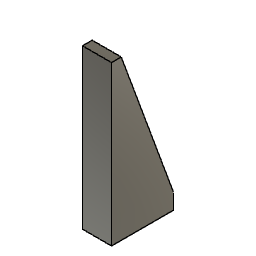
Front Panel Holders v2 (Autodesk Fusion 360 design; units mm, degrees)
Autodesk Fusion 360 part; units mm, degrees
sketch "Sketch1" plane through (0, 0, 0) normal (0, 1, 0) x (1, 0, 0)
  line L0 (0, 0) -> (15, 0)
  line L1 (15, 0) -> (15, -80)
  line L2 (15, -80) -> (0, -80)
  line L3 (0, -80) -> (0, 0)
  dimension "d4" = 15
  dimension "d5" = 80
  constraint horizontal L0
  constraint vertical L1
  constraint horizontal L2
  constraint vertical L3
  constraint coincident L0.start L3.end
  measures "d4" distance of L0.start L0.end
  measures "d5" distance of L0.start L2.end
extrude "Extrude1" add sketch "Sketch1" along normal blind 5
sketch "Sketch3" plane through (0, 5, 0) normal (0, 1, 0) x (-1, 0, 0)
  line L0 (0, 80) -> (-15, 80)
  line L1 (-15, 80) -> (-15, 0)
  line L2 (-15, 0) -> (0, 0)
  line L3 (0, 0) -> (0, 80)
  line L4 (-15, 0) -> (-10, 0)
  line L5 (-10, 0) -> (-10, 8)
  line L6 (-10, 8) -> (-15, 8)
  line L7 (-15, 8) -> (-15, 0)
  dimension "d10" = 5
  dimension "d11" = 8
  constraint horizontal L4
  constraint vertical L5
  constraint horizontal L6
  constraint vertical L7
  constraint coincident L1.end L2.start
  measures "d10" distance of L1.end L4.end
  measures "d11" distance of L1.end L6.end
extrude "Extrude2" add sketch "Sketch3" along normal blind 35 contours L1 L2 L4 L5 L6 L7
sketch "Sketch4" plane through (15, 0, 0) normal (1, 0, 0) x (0, 1, 0)
  line L0 (0, 80) -> (0, 0)
  line L1 (0, 0) -> (40, 0)
  line L2 (40, 0) -> (40, 8)
  line L3 (40, 8) -> (5, 8)
  line L4 (5, 8) -> (5, 80)
  line L5 (5, 80) -> (0, 80)
  line L6 (5, 80) -> (40, 8)
  line L7 (40, 8) -> (5, 8)
  line L8 (5, 8) -> (5, 80)
  constraint coincident L4.end L5.start
  constraint coincident L2.end L3.start
  constraint coincident L3.end L4.start
extrude "Extrude4" add 1 faces at (10, 1.6667, 80) along direction (0, 0, 1) blind 2
extrude "Extrude6" cut 1 faces at (13.3333, 40, 5.3333) along direction (0, -1, 0) blind 8
sketch "Sketch6" plane through (15, 0, 0) normal (1, 0, 0) x (0, 1, 0)
  line L0 (32, 0) -> (32, 8)
  line L1 (32, 8) -> (5, 8)
  line L2 (5, 8) -> (5, 82)
  line L3 (5, 82) -> (0, 82)
  line L4 (0, 82) -> (0, 0)
  line L5 (0, 0) -> (32, 0)
  line L6 (5, 82) -> (5, 8)
  line L7 (5, 8) -> (32, 8)
  line L8 (32, 8) -> (5, 82)
  constraint coincident L2.end L3.start
  constraint coincident L1.end L2.start
  constraint coincident L0.end L1.start
extrude "Extrude7" add sketch "Sketch6" against normal blind 5 contours L1 L2 L6 L7 L8
sketch "Sketch7" plane through (0, 0, 0) normal (0, 0, -1) x (1, 0, 0)
  line L0 (10, -32) -> (15, -32)
  line L1 (15, -32) -> (15, 0)
  line L2 (15, 0) -> (0, 0)
  line L3 (0, 0) -> (0, -5)
  line L4 (0, -5) -> (10, -5)
  line L5 (10, -5) -> (10, -32)
  line L6 (10, -32) -> (10, -5)
  line L7 (10, -5) -> (0, -5)
  line L8 (0, -5) -> (10, -32)
  constraint coincident L0.start L5.end
  constraint coincident L4.end L5.start
  constraint coincident L3.end L4.start
extrude "Extrude8" add sketch "Sketch7" against normal blind 3 contours L4 L5 L6 L7 L8
